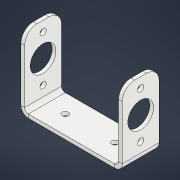
# Autodesk Inventor part: Flat Pattern
Saved by Autodesk Inventor 2022 (Build 260153000, 153)
## iProperties
Created: 2021-10-05
Part Number: Flat Pattern
Material: Generic
Document SubType Name: Sheet Metal
Designer: Administrator
Density: 1 g/cm^3
Appearance: Default
Sheet Metal Rule: 0.08in
Sheet Metal Width: 0.000 mm
Sheet Metal Length: 0.000 mm
Sheet Metal Area: 0.000 mm^2
Title: Flat Pattern
Author: Administrator
Autodesk Inventor part; units mm, degrees
ref_plane "YZ Plane" through (0, 0, 0) normal (1, 0, 0) x (0, 1, 0)
ref_plane "XZ Plane" through (0, 0, 0) normal (0, 1, 0) x (-1, 0, 0)
ref_plane "XY Plane" through (0, 0, 0) normal (0, 0, 1) x (1, 0, 0)
sketch "Sketch3" plane through (0, 0, 0) normal (0, 1, 0) x (-1, 0, 0)
  line L0 (55, 0) -> (0, 0)
  line L1 (0, 0) -> (0, -20)
  line L2 (0, -20) -> (55, -20)
  line L3 (55, -20) -> (55, 0)
  dimension "d9" = 55
  dimension "d10" = 20
  measures "d9" distance of L0.start L0.end
  measures "d10" distance of L0.end L1.end
extrude "Plate1" add sketch "Sketch3" along normal blind 2.032
sketch "Sketch4" plane through (-52.968, 0, 0) normal (-1, 0, 0) x (0, -1, 0)
  line L0 (0, -20) -> (0, 0)
  line L1 (0, 0) -> (-40, 0)
  line L2 (-40, 0) -> (-40, -20)
  line L3 (-40, -20) -> (0, -20)
  constraints: 6 end point, 1 horizontal, 1 perpendicular, 1 vertical
edge flange "Flange1" height 40 angle 90 thickness 2.032 bend radius 2.032 thickness toward (-1, 0, 0) relief straight relief width 2.032 relief depth 1.016 corner gap 2.032 corner form 0 edges at (-55, 2.032, -10) (0, 2.032, -10) wall of the first edge with corners at (-52.968, 0, -20) (-52.968, 0, 0) (-52.968, 40, 0) (-52.968, 40, -20)
bend "Bend1"
corner "Corner1"
sketch "Sketch5" plane through (0, 40, 0) normal (1, 0, 0) x (0, 0, -1)
  line L0 (0, -35.936) -> (20, -35.936) projected
  line L1 (0, -35.936) -> (20, -35.936) projected
  line L2 (20, 0) -> (20, -35.936) projected
  line L3 (0, 0) -> (20, 0) projected
  line L4 (0, -35.936) -> (0, 0) projected
  line L5 (20, -35.936) -> (20, 0) projected
  line L6 (20, -17.968) -> (0, -17.968) construction
  line L7 (0, -35.936) -> (0, 0) projected
  point P0 (0, -40)
  point P1 (10, -5.468)
  point P2 (10, -17.968)
  point P3 (10, -30.468)
  point P4 (10, -35.936)
  point P5 (10, -17.968)
  dimension "d22" = 12.5
  dimension "d23" = 12.5
  constraints: 4 midpoint, 3 vertical alignment, 2 end point, 1 coincident
  measures "d22" distance of point (10, -30.468) point (10, -17.968)
  measures "d23" distance of point (10, -5.468) point (10, -17.968)
hole "Hole1" at (0, 9.532, -10) at (0, 34.532, -10) direction (-1, 0, 0) diameter 3.4 depth 55 tip angle 118 clearance for "Socket Head Cap Screw" size "M3" standard "Ansi Metric M Profile"
hole "Hole2" at (0, 22.032, -10) direction (-1, 0, 0) diameter 14 depth 55 tip angle 118
fillet "Fillet1" radius 6.7625 4 edges at (-53.984, 40, -20) (-53.984, 40, 0) (-1.016, 40, 0) (-1.016, 40, -20)
sketch "Sketch6" plane through (0, 2.032, 0) normal (0, 1, 0) x (1, 0, 0)
  line L0 (-4.064, 0) -> (-4.064, 20) projected
  line L1 (-50.936, 20) -> (-4.064, 20) projected
  line L2 (-50.936, 20) -> (-50.936, 0) projected
  line L3 (-4.064, 0) -> (-50.936, 0) projected
  line L4 (-4.064, 0) -> (-4.064, 20) projected
  line L5 (-4.064, 10) -> (-14.064, 10) construction
  line L6 (-40.936, 10) -> (-50.936, 10) construction
  point P0 (0, 0)
  dimension "d39" = 10
  constraints: 4 end point, 2 horizontal, 2 midpoint, 1 collinear
  measures "d39" distance of L6.start L6.end
hole "Hole3" at (-40.936, 2.032, -10) at (-14.064, 2.032, -10) direction (0, -1, 0) diameter 3.4 end through all clearance for "Socket Head Cap Screw" size "M3" standard "Ansi Metric M Profile"
equation "\"d29\" = Thickness"
equation "\"d11\" = Thickness"
equation "\"d12\" = BendReliefWidth"
equation "\"d13\" = BendReliefDepth"
equation "\"d14\" = MinimumRemnant"
equation "\"d15\" = TransitionRadius"
equation "\"d18\" = BendRadius"
equation "\"d19\" = CornerReliefSize"
equation "\"d20\" = GapSize"
equation "\"d21\" = JacobiRadiusSize"
equation "\"BendRadius\" = Thickness"
equation "\"BendReliefWidth\" = Thickness"
equation "\"BendReliefDepth\" = 0.5 * Thickness"
equation "\"CornerReliefSize\" = 4 * Thickness"
equation "\"MinimumRemnant\" = 2 * Thickness"
equation "\"TransitionRadius\" = BendRadius"
equation "\"JacobiRadiusSize\" = BendRadius"
equation "\"GapSize\" = Thickness"
equation "\"Thickness\" = 2.032"
body "Solid5"
